Autodesk Inventor part; units mm, degrees
(part 2 of 3)
  line L1096 (95.9721, -65) -> (95.9721, -70)
  line L1097 (107.9721, -65) -> (102.9721, -65)
  line L1098 (100.9721, -70) -> (100.9721, -65)
  line L1099 (102.9721, -65) -> (102.9721, -70)
  line L1100 (107.9721, -70) -> (107.9721, -65)
  line L1101 (102.9721, -70) -> (107.9721, -70)
  line L1102 (114.9721, -65) -> (109.9721, -65)
  line L1103 (109.9721, -65) -> (109.9721, -70)
  line L1104 (109.9721, -70) -> (114.9721, -70)
  line L1105 (114.9721, -70) -> (114.9721, -65)
  line L1106 (116.9721, -65) -> (116.9721, -70)
  line L1107 (128.9721, -65) -> (123.9721, -65)
  line L1108 (128.9721, -70) -> (128.9721, -65)
  line L1109 (123.9721, -70) -> (128.9721, -70)
  line L1110 (121.9721, -65) -> (116.9721, -65)
  line L1111 (121.9721, -70) -> (121.9721, -65)
  line L1112 (116.9721, -70) -> (121.9721, -70)
  line L1113 (123.9721, -65) -> (123.9721, -70)
  line L1114 (142.9721, -65) -> (137.9721, -65)
  line L1115 (137.9721, -70) -> (142.9721, -70)
  line L1116 (142.9721, -70) -> (142.9721, -65)
  line L1117 (137.9721, -65) -> (137.9721, -70)
  line L1118 (135.9721, -65) -> (130.9721, -65)
  line L1119 (135.9721, -70) -> (135.9721, -65)
  line L1120 (130.9721, -65) -> (130.9721, -70)
  line L1121 (130.9721, -70) -> (135.9721, -70)
  line L1122 (156.9721, -14) -> (156.9721, -9)
  line L1123 (156.9721, -9) -> (151.9721, -9)
  line L1124 (151.9721, -14) -> (156.9721, -14)
  line L1125 (151.9721, -9) -> (151.9721, -14)
  line L1126 (156.9721, -16) -> (151.9721, -16)
  line L1127 (151.9721, -21) -> (156.9721, -21)
  line L1128 (156.9721, -21) -> (156.9721, -16)
  line L1129 (151.9721, -16) -> (151.9721, -21)
  line L1130 (151.9721, -23) -> (151.9721, -28)
  line L1131 (156.9721, -23) -> (151.9721, -23)
  line L1132 (151.9721, -28) -> (156.9721, -28)
  line L1133 (156.9721, -28) -> (156.9721, -23)
  line L1134 (151.9721, -30) -> (151.9721, -35)
  line L1135 (156.9721, -30) -> (151.9721, -30)
  line L1136 (151.9721, -35) -> (156.9721, -35)
  line L1137 (156.9721, -35) -> (156.9721, -30)
  line L1138 (151.9721, -37) -> (151.9721, -42)
  line L1139 (156.9721, -37) -> (151.9721, -37)
  line L1140 (151.9721, -42) -> (156.9721, -42)
  line L1141 (156.9721, -42) -> (156.9721, -37)
  line L1142 (151.9721, -44) -> (151.9721, -49)
  line L1143 (156.9721, -44) -> (151.9721, -44)
  line L1144 (151.9721, -49) -> (156.9721, -49)
  line L1145 (156.9721, -49) -> (156.9721, -44)
  line L1146 (151.9721, -51) -> (151.9721, -56)
  line L1147 (156.9721, -51) -> (151.9721, -51)
  line L1148 (151.9721, -56) -> (156.9721, -56)
  line L1149 (156.9721, -56) -> (156.9721, -51)
  line L1150 (163.9721, -14) -> (163.9721, -9)
  line L1151 (163.9721, -9) -> (158.9721, -9)
  line L1152 (158.9721, -9) -> (158.9721, -14)
  line L1153 (158.9721, -14) -> (163.9721, -14)
  line L1154 (163.9721, -16) -> (158.9721, -16)
  line L1155 (158.9721, -21) -> (163.9721, -21)
  line L1156 (163.9721, -21) -> (163.9721, -16)
  line L1157 (158.9721, -16) -> (158.9721, -21)
  line L1158 (163.9721, -23) -> (158.9721, -23)
  line L1159 (158.9721, -23) -> (158.9721, -28)
  line L1160 (158.9721, -28) -> (163.9721, -28)
  line L1161 (163.9721, -28) -> (163.9721, -23)
  line L1162 (163.9721, -30) -> (158.9721, -30)
  line L1163 (158.9721, -30) -> (158.9721, -35)
  line L1164 (158.9721, -35) -> (163.9721, -35)
  line L1165 (163.9721, -35) -> (163.9721, -30)
  line L1166 (158.9721, -44) -> (158.9721, -49)
  line L1167 (163.9721, -49) -> (163.9721, -44)
  line L1168 (163.9721, -44) -> (158.9721, -44)
  line L1169 (158.9721, -42) -> (163.9721, -42)
  line L1170 (163.9721, -42) -> (163.9721, -37)
  line L1171 (163.9721, -37) -> (158.9721, -37)
  line L1172 (158.9721, -37) -> (158.9721, -42)
  line L1173 (158.9721, -49) -> (163.9721, -49)
  line L1174 (172.9721, -9) -> (172.9721, -14)
  line L1175 (172.9721, -14) -> (177.9721, -14)
  line L1176 (177.9721, -14) -> (177.9721, -9)
  line L1177 (177.9721, -9) -> (172.9721, -9)
  line L1178 (109.9721, 65) -> (114.9721, 65)
  line L1179 (116.9721, 65) -> (121.9721, 65)
  line L1180 (114.9721, 70) -> (109.9721, 70)
  line L1181 (114.9721, 65) -> (114.9721, 70)
  line L1182 (116.9721, 70) -> (116.9721, 65)
  line L1183 (121.9721, 70) -> (116.9721, 70)
  line L1184 (121.9721, 65) -> (121.9721, 70)
  line L1185 (109.9721, 70) -> (109.9721, 65)
  line L1186 (107.9721, 65) -> (107.9721, 70)
  line L1187 (102.9721, 65) -> (107.9721, 65)
  line L1188 (107.9721, 70) -> (102.9721, 70)
  line L1189 (102.9721, 70) -> (102.9721, 65)
  line L1190 (88.9721, 65) -> (93.9721, 65)
  line L1191 (95.9721, 70) -> (95.9721, 65)
  line L1192 (100.9721, 70) -> (95.9721, 70)
  line L1193 (93.9721, 65) -> (93.9721, 70)
  line L1194 (93.9721, 70) -> (88.9721, 70)
  line L1195 (100.9721, 65) -> (100.9721, 70)
  line L1196 (95.9721, 65) -> (100.9721, 65)
  line L1197 (88.9721, 70) -> (88.9721, 65)
  line L1198 (86.9721, 65) -> (86.9721, 70)
  line L1199 (81.9721, 65) -> (86.9721, 65)
  line L1200 (81.9721, 70) -> (81.9721, 65)
  line L1201 (86.9721, 70) -> (81.9721, 70)
  line L1202 (67.9721, 65) -> (72.9721, 65)
  line L1203 (67.9721, 70) -> (67.9721, 65)
  line L1204 (72.9721, 70) -> (67.9721, 70)
  line L1205 (74.9721, 65) -> (79.9721, 65)
  line L1206 (72.9721, 65) -> (72.9721, 70)
  line L1207 (74.9721, 70) -> (74.9721, 65)
  line L1208 (79.9721, 65) -> (79.9721, 70)
  line L1209 (79.9721, 70) -> (74.9721, 70)
  line L1210 (123.9721, 65) -> (128.9721, 65)
  line L1211 (128.9721, 70) -> (123.9721, 70)
  line L1212 (123.9721, 70) -> (123.9721, 65)
  line L1213 (128.9721, 65) -> (128.9721, 70)
  line L1214 (130.9721, 65) -> (135.9721, 65)
  line L1215 (130.9721, 70) -> (130.9721, 65)
  line L1216 (135.9721, 65) -> (135.9721, 70)
  line L1217 (137.9721, 70) -> (137.9721, 65)
  line L1218 (135.9721, 70) -> (130.9721, 70)
  line L1219 (137.9721, 65) -> (142.9721, 65)
  line L1220 (142.9721, 70) -> (137.9721, 70)
  line L1221 (142.9721, 65) -> (142.9721, 70)
  line L1222 (53.9721, 70) -> (53.9721, 65)
  line L1223 (58.9721, 70) -> (53.9721, 70)
  line L1224 (53.9721, 65) -> (58.9721, 65)
  line L1225 (58.9721, 65) -> (58.9721, 70)
  line L1226 (60.9721, 70) -> (60.9721, 65)
  line L1227 (65.9721, 70) -> (60.9721, 70)
  line L1228 (60.9721, 65) -> (65.9721, 65)
  line L1229 (65.9721, 65) -> (65.9721, 70)
  line L1230 (39.9721, 70) -> (39.9721, 65)
  line L1231 (44.9721, 70) -> (39.9721, 70)
  line L1232 (44.9721, 65) -> (44.9721, 70)
  line L1233 (46.9721, 70) -> (46.9721, 65)
  line L1234 (46.9721, 65) -> (51.9721, 65)
  line L1235 (51.9721, 65) -> (51.9721, 70)
  line L1236 (51.9721, 70) -> (46.9721, 70)
  line L1237 (39.9721, 65) -> (44.9721, 65)
  line L1238 (102.9721, 77) -> (102.9721, 72)
  line L1239 (100.9721, 72) -> (100.9721, 77)
  line L1240 (95.9721, 72) -> (100.9721, 72)
  line L1241 (100.9721, 77) -> (95.9721, 77)
  line L1242 (93.9721, 77) -> (88.9721, 77)
  line L1243 (93.9721, 72) -> (93.9721, 77)
  line L1244 (95.9721, 77) -> (95.9721, 72)
  line L1245 (88.9721, 72) -> (93.9721, 72)
  line L1246 (88.9721, 77) -> (88.9721, 72)
  line L1247 (81.9721, 72) -> (86.9721, 72)
  line L1248 (86.9721, 72) -> (86.9721, 77)
  line L1249 (86.9721, 77) -> (81.9721, 77)
  line L1250 (72.9721, 72) -> (72.9721, 77)
  line L1251 (74.9721, 77) -> (74.9721, 72)
  line L1252 (79.9721, 77) -> (74.9721, 77)
  line L1253 (79.9721, 72) -> (79.9721, 77)
  line L1254 (81.9721, 77) -> (81.9721, 72)
  line L1255 (74.9721, 72) -> (79.9721, 72)
  line L1256 (67.9721, 77) -> (67.9721, 72)
  line L1257 (72.9721, 77) -> (67.9721, 77)
  line L1258 (67.9721, 72) -> (72.9721, 72)
  line L1259 (65.9721, 72) -> (65.9721, 77)
  line L1260 (60.9721, 72) -> (65.9721, 72)
  line L1261 (60.9721, 77) -> (60.9721, 72)
  line L1262 (65.9721, 77) -> (60.9721, 77)
  line L1263 (58.9721, 77) -> (53.9721, 77)
  line L1264 (58.9721, 72) -> (58.9721, 77)
  line L1265 (53.9721, 72) -> (58.9721, 72)
  line L1266 (53.9721, 77) -> (53.9721, 72)
  line L1267 (123.9721, 72) -> (128.9721, 72)
  line L1268 (128.9721, 77) -> (123.9721, 77)
  line L1269 (123.9721, 77) -> (123.9721, 72)
  line L1270 (116.9721, 72) -> (121.9721, 72)
  line L1271 (121.9721, 72) -> (121.9721, 77)
  line L1272 (121.9721, 77) -> (116.9721, 77)
  line L1273 (116.9721, 77) -> (116.9721, 72)
  line L1274 (114.9721, 72) -> (114.9721, 77)
  line L1275 (109.9721, 72) -> (114.9721, 72)
  line L1276 (114.9721, 77) -> (109.9721, 77)
  line L1277 (102.9721, 72) -> (107.9721, 72)
  line L1278 (109.9721, 77) -> (109.9721, 72)
  line L1279 (107.9721, 72) -> (107.9721, 77)
  line L1280 (107.9721, 77) -> (102.9721, 77)
  line L1281 (128.9721, 72) -> (128.9721, 77)
  line L1282 (109.9721, 79) -> (114.9721, 79)
  line L1283 (114.9721, 79) -> (114.9721, 84)
  line L1284 (114.9721, 84) -> (109.9721, 84)
  line L1285 (102.9721, 79) -> (107.9721, 79)
  line L1286 (107.9721, 79) -> (107.9721, 84)
  line L1287 (102.9721, 84) -> (102.9721, 79)
  line L1288 (107.9721, 84) -> (102.9721, 84)
  line L1289 (109.9721, 84) -> (109.9721, 79)
  line L1290 (88.9721, 79) -> (93.9721, 79)
  line L1291 (93.9721, 84) -> (88.9721, 84)
  line L1292 (95.9721, 79) -> (100.9721, 79)
  line L1293 (93.9721, 79) -> (93.9721, 84)
  line L1294 (95.9721, 84) -> (95.9721, 79)
  line L1295 (100.9721, 84) -> (95.9721, 84)
  line L1296 (100.9721, 79) -> (100.9721, 84)
  line L1297 (81.9721, 79) -> (86.9721, 79)
  line L1298 (88.9721, 84) -> (88.9721, 79)
  line L1299 (86.9721, 79) -> (86.9721, 84)
  line L1300 (86.9721, 84) -> (81.9721, 84)
  line L1301 (81.9721, 84) -> (81.9721, 79)
  line L1302 (67.9721, 84) -> (67.9721, 79)
  line L1303 (72.9721, 84) -> (67.9721, 84)
  line L1304 (67.9721, 79) -> (72.9721, 79)
  line L1305 (74.9721, 79) -> (79.9721, 79)
  line L1306 (72.9721, 79) -> (72.9721, 84)
  line L1307 (79.9721, 84) -> (74.9721, 84)
  line L1308 (79.9721, 79) -> (79.9721, 84)
  line L1309 (74.9721, 84) -> (74.9721, 79)
  line L1310 (170.9721, -14) -> (170.9721, -9)
  line L1311 (170.9721, -21) -> (170.9721, -16)
  line L1312 (165.9721, -14) -> (170.9721, -14)
  line L1313 (165.9721, -9) -> (165.9721, -14)
  line L1314 (170.9721, -16) -> (165.9721, -16)
  line L1315 (170.9721, -9) -> (165.9721, -9)
  line L1316 (165.9721, -16) -> (165.9721, -21)
  line L1317 (165.9721, -23) -> (165.9721, -28)
  line L1318 (170.9721, -28) -> (170.9721, -23)
  line L1319 (170.9721, -23) -> (165.9721, -23)
  line L1320 (165.9721, -21) -> (170.9721, -21)
  line L1321 (165.9721, -30) -> (165.9721, -35)
  line L1322 (165.9721, -28) -> (170.9721, -28)
  line L1323 (170.9721, -30) -> (165.9721, -30)
  line L1324 (165.9721, -35) -> (170.9721, -35)
  line L1325 (170.9721, -35) -> (170.9721, -30)
  line L1326 (121.9721, -72) -> (116.9721, -72)
  line L1327 (116.9721, -77) -> (121.9721, -77)
  line L1328 (121.9721, -77) -> (121.9721, -72)
  line L1329 (123.9721, -72) -> (123.9721, -77)
  line L1330 (128.9721, -72) -> (123.9721, -72)
  line L1331 (128.9721, -77) -> (128.9721, -72)
  line L1332 (123.9721, -77) -> (128.9721, -77)
  line L1333 (114.9721, -72) -> (109.9721, -72)
  line L1334 (109.9721, -77) -> (114.9721, -77)
  line L1335 (114.9721, -77) -> (114.9721, -72)
  line L1336 (116.9721, -72) -> (116.9721, -77)
  line L1337 (100.9721, -77) -> (100.9721, -72)
  line L1338 (107.9721, -72) -> (102.9721, -72)
  line L1339 (102.9721, -72) -> (102.9721, -77)
  line L1340 (102.9721, -77) -> (107.9721, -77)
  line L1341 (107.9721, -77) -> (107.9721, -72)
  line L1342 (109.9721, -72) -> (109.9721, -77)
  line L1343 (95.9721, -77) -> (100.9721, -77)
  line L1344 (95.9721, -72) -> (95.9721, -77)
  line L1345 (100.9721, -72) -> (95.9721, -72)
  line L1346 (114.9721, -84) -> (114.9721, -79)
  line L1347 (114.9721, -79) -> (109.9721, -79)
  line L1348 (109.9721, -84) -> (114.9721, -84)
  line L1349 (107.9721, -79) -> (102.9721, -79)
  line L1350 (109.9721, -79) -> (109.9721, -84)
  line L1351 (107.9721, -84) -> (107.9721, -79)
  line L1352 (102.9721, -84) -> (107.9721, -84)
  line L1353 (102.9721, -79) -> (102.9721, -84)
  line L1354 (100.9721, -84) -> (100.9721, -79)
  line L1355 (100.9721, -79) -> (95.9721, -79)
  line L1356 (95.9721, -84) -> (100.9721, -84)
  line L1357 (95.9721, -79) -> (95.9721, -84)
  dimension "d613" = 2
  dimension "d614" = 5
  dimension "d615" = 5
  dimension "d616" = 82
  dimension "d619" = 7
  dimension "d626" = 7
  dimension "d633" = 7
  dimension "d640" = 7
  dimension "d647" = 7
  dimension "d654" = 7
  dimension "d682" = 9
  dimension "d689" = 7
  dimension "d696" = 7
  dimension "d717" = 7
  dimension "d724" = 7
  dimension "d738" = 7
  dimension "d748" = 7
  dimension "d755" = 7
  dimension "d762" = 7
  dimension "d769" = 7
  dimension "d776" = 7
  dimension "d783" = 7
  constraints: 2712 end point, 14 vertical, 5 horizontal, 2 parallel, 1 perpendicular, 2704 other
  measures "d613" distance between parallel lines of L4 L0
  measures "d614" distance between parallel lines of L2 L0
  measures "d615" distance between parallel lines of L3 L1
  measures "d616" distance between parallel lines of L5 L1
  measures "d619" distance of L0.start L6.start
  measures "d626" distance of L0.start L102.start
  measures "d633" distance of L22.start L110.end
  measures "d640" distance of L400.end L481.end
  measures "d647" distance of L574.start L646.start
  measures "d654" distance of L677.start L724.start
  measures "d682" distance of L62.start L796.start
  measures "d689" distance of L834.end L838.end
  measures "d696" distance of L1081.start L1094.start
  measures "d717" distance of L839.start L1122.end
  measures "d724" distance of L1122.end L1150.end
  measures "d738" distance of L812.end L1174.end
  measures "d748" distance of L739.end L1178.end
  measures "d755" distance of L1187.start L1238.end
  measures "d762" distance of L1274.start L1282.end
  measures "d769" distance of L1150.end L1310.end
  measures "d776" distance of L1110.start L1326.start
  measures "d783" distance of L1333.start L1346.end
extrude "Выдавливание103" cut sketch "Эскиз119" against normal blind 10
sketch "Эскиз120" plane through (-91.9721, 4, 0) normal (0, 1, 0) x (1, 0, 0)
  line L0 (-43.9191, 0) -> (225.9723, 0)
  line L1 (225.9723, 0) -> (225.9723, -109.5505)
  line L2 (225.9723, -109.5505) -> (-43.9191, -109.5505)
  line L3 (-43.9191, -109.5505) -> (-43.9191, 0)
  point P0 (91.9721, 0)
  constraints: 8 end point, 2 parallel, 1 horizontal, 1 perpendicular
extrude "Выдавливание104" cut sketch "Эскиз120" against normal through all
mirror "Зеркальное отражение8" about plane through (-46.203, 1.9857, 0) normal (0, 0, 1)
sketch "Эскиз121" plane through (0, 0, 0) normal (0, -1, 0) x (1, 0, 0)
  line L0 (-10, -10) -> (10, -10)
  line L1 (10, -10) -> (10, 10)
  line L2 (10, 10) -> (-10, 10)
  line L3 (-10, 10) -> (-10, -10)
  line L4 (-10, -10) -> (10, 10) construction
  line L5 (10, -10) -> (-10, 10) construction
  point P0 (0, 0)
  dimension "d790" = 20
  dimension "d791" = 20
  constraints: 12 end point, 2 collinear, 2 midpoint, 1 perpendicular, 1 vertical
  measures "d790" distance of L2.end L1.end
  measures "d791" distance of L1.end L0.end
extrude "Выдавливание105" add sketch "Эскиз121" against normal up to surface (4 mm away)
extrude "Выдавливание106" add sketch "Эскиз121" along normal blind 5
sketch "Эскиз122" plane through (0, -5, 0) normal (0, -1, 0) x (1, 0, 0)
  line L0 (-7.5, -7.5) -> (7.5, -7.5)
  line L1 (7.5, -7.5) -> (7.5, 7.5)
  line L2 (7.5, 7.5) -> (-7.5, 7.5)
  line L3 (-7.5, 7.5) -> (-7.5, -7.5)
  line L4 (-7.5, -7.5) -> (7.5, 7.5) construction
  line L5 (7.5, -7.5) -> (-7.5, 7.5) construction
  point P0 (0, 0)
  dimension "d796" = 15
  dimension "d797" = 15
  dimension "d12" = 100
  dimension "d14" = 17
  dimension "d26" = 5
  constraints: 12 end point, 2 midpoint, 2 parallel, 1 horizontal, 1 perpendicular
  measures "d796" distance of L2.end L1.end
  measures "d797" distance of L1.end L0.end
extrude "Выдавливание107" cut sketch "Эскиз122" against normal blind 3
sketch "Эскиз6" plane through (0, -35, -85) normal (0, -1, 0) x (1, 0, 0)
  arc A0 (29.3991, 164.4544) -> (0, 170) centre (-5, 62.7941) ccw projected
  line L0 (0, 170) -> (0, 0) projected
  arc A1 (0, 0) -> (29.3991, 5.5456) centre (-5, 107.2059) ccw projected
  arc A2 (29.3991, 5.5456) -> (100, 85) centre (-5, 107.2059) ccw projected
  arc A3 (100, 85) -> (29.3991, 164.4544) centre (-5, 62.7941) ccw projected
  point P0 (0, 85)
  dimension "d121" = 143.8029
  constraints: 4 end point, 2 point on circle, 1 centre point, 1 coincident, 1 horizontal, 1 vertical
  measures "d121" radius of A0
sketch "Эскиз26" plane through (0, -165, -85) normal (0, -1, 0) x (1, 0, 0)
  arc A0 (97.9549, 85) -> (2, 167.8837) centre (-5, 62.7941) ccw projected
  line L0 (97.9395, 85) -> (97.9395, 85) construction
  line L1 (32, 161.4035) -> (32, 85)
  line L2 (2, 85) -> (100, 85) construction
  line L3 (2, 0.112) -> (2, 167.8837) construction
  line L4 (34, 160.6298) -> (34, 85)
  line L5 (32, 85) -> (34, 85)
  point P0 (0, 85)
  point P1 (2, 22)
  dimension "d144" = 30
  dimension "d145" = 2
  constraints: 6 end point, 2 point on circle, 2 point on line, 1 horizontal, 1 perpendicular, 1 vertical
  measures "d144" distance between parallel lines of L1 L3
  measures "d145" distance between parallel lines of L4 L1
sketch "Эскиз28" plane through (34, -165, 75.6298) normal (1, 0, 0) x (0, 0, -1)
  circle A0 centre (68.6298, 7) radius 5 projected
  line L0 (75.6298, 0) -> (75.6298, 230.325) projected
  line L1 (75.6298, 0) -> (-0.7738, 0) projected
  line L2 (75.6298, 14) -> (61.6298, 14) construction
  line L3 (61.6298, 14) -> (61.6298, 0) construction
  line L4 (160.5178, 0) -> (-7.2539, 0) projected
  line L5 (72.6298, 17) -> (65.6298, 17)
  line L6 (65.6298, 17) -> (65.6298, 27)
  line L7 (65.6298, 27) -> (72.6298, 27)
  line L8 (72.6298, 27) -> (72.6298, 17)
  point P0 (75.6298, 165)
  point P1 (138.6298, 0)
  dimension "d156" = 14
  dimension "d157" = 14
  dimension "d158" = 7
  dimension "d159" = 10
  dimension "d160" = 3
  dimension "d161" = 3
  constraints: 12 end point, 2 horizontal, 2 parallel, 2 perpendicular, 2 point on line
  measures "d156" distance of L0.start L2.start
  measures "d157" distance of L2.start L2.end
  measures "d158" distance of L6.end L7.end
  measures "d159" distance of L5.end L6.end
  measures "d160" distance between parallel lines of L2 L5
  measures "d161" distance between parallel lines of L0 L8
sketch "Эскиз29" plane through (34, -165, 75.6298) normal (1, 0, 0) x (0, 0, -1)
  circle A0 centre (68.6298, 7) radius 5 projected
  line L0 (75.6298, 0) -> (-0.7738, 0) projected
  line L1 (75.6298, 0) -> (75.6298, 230.325) projected
  line L2 (75.6298, 14) -> (61.6298, 14)
  line L3 (61.6298, 14) -> (61.6298, 0)
  line L4 (-9.3702, 0) -> (160.6298, 0) projected
  line L5 (58.6298, 2) -> (51.6298, 2)
  line L6 (51.6298, 2) -> (51.6298, 12)
  line L7 (51.6298, 12) -> (58.6298, 12)
  line L8 (58.6298, 12) -> (58.6298, 2)
  line L9 (65.6298, 17) -> (72.6298, 17) projected
  point P0 (75.6298, 165)
  dimension "d164" = 14
  dimension "d165" = 14
  dimension "d166" = 3
  dimension "d167" = 2
  dimension "d168" = 7
  dimension "d169" = 10
  constraints: 12 end point, 2 horizontal, 2 parallel, 2 perpendicular, 2 point on line
  measures "d164" distance of L2.end L3.end
  measures "d165" distance of L2.start L2.end
  measures "d166" distance between parallel lines of L3 L8
  measures "d167" distance between parallel lines of L0 L5
  measures "d168" distance of L6.end L7.end
  measures "d169" distance of L6.end L5.end
sketch "Эскиз30" plane through (34, -165, 75.6298) normal (1, 0, 0) x (0, 0, -1)
  line L0 (51.6298, 12) -> (51.6298, 2) projected
  line L1 (58.6298, 12) -> (51.6298, 12) projected
  line L2 (58.6298, 2) -> (58.6298, 12) projected
  line L3 (51.6298, 2) -> (58.6298, 2) projected
  line L4 (39.6298, 12) -> (39.6298, 2)
  line L5 (46.6298, 12) -> (39.6298, 12)
  line L6 (46.6298, 2) -> (46.6298, 12)
  line L7 (39.6298, 2) -> (46.6298, 2)
  point P0 (75.6298, 165)
  point P1 (43.1298, 2)
  dimension "d178" = 7
  dimension "d179" = 10
  dimension "d180" = 5
  constraints: 8 end point, 1 horizontal, 1 horizontal alignment, 1 midpoint, 1 vertical
  measures "d178" distance between parallel lines of L4 L6
  measures "d179" distance between parallel lines of L7 L5
  measures "d180" distance between parallel lines of L6 L0
sketch "Эскиз31" plane through (34, -165, 75.6298) normal (1, 0, 0) x (0, 0, -1)
  line L0 (46.6298, 12) -> (39.6298, 12) projected
  line L1 (39.6298, 12) -> (39.6298, 2) projected
  line L2 (46.6298, 2) -> (46.6298, 12) projected
  line L3 (39.6298, 2) -> (46.6298, 2) projected
  line L4 (34.6298, 12) -> (27.6298, 12)
  line L5 (27.6298, 12) -> (27.6298, 2)
  line L6 (34.6298, 2) -> (34.6298, 12)
  line L7 (27.6298, 2) -> (34.6298, 2)
  point P0 (75.6298, 165)
  dimension "d186" = 10
  dimension "d187" = 7
  dimension "d188" = 5
  constraints: 8 end point, 2 horizontal, 2 vertical, 1 horizontal alignment
  measures "d186" distance of L6.start L4.start
  measures "d187" distance of L4.start L4.end
  measures "d188" distance between parallel lines of L1 L6
sketch "Эскиз32" plane through (34, -165, 75.6298) normal (1, 0, 0) x (0, 0, -1)
  line L0 (34.6298, 12) -> (27.6298, 12) projected
  line L1 (27.6298, 12) -> (27.6298, 2) projected
  line L2 (34.6298, 2) -> (34.6298, 12) projected
  line L3 (27.6298, 2) -> (34.6298, 2) projected
  line L4 (22.6298, 12) -> (15.6298, 12)
  line L5 (15.6298, 12) -> (15.6298, 2)
  line L6 (22.6298, 2) -> (22.6298, 12)
  line L7 (15.6298, 2) -> (22.6298, 2)
  point P0 (75.6298, 165)
  dimension "d194" = 10
  dimension "d195" = 7
  dimension "d196" = 5
  constraints: 8 end point, 2 horizontal, 2 vertical, 1 horizontal alignment
  measures "d194" distance of L6.start L4.start
  measures "d195" distance of L4.start L4.end
  measures "d196" distance between parallel lines of L6 L1
sketch "Эскиз33" plane through (34, -165, 75.6298) normal (1, 0, 0) x (0, 0, -1)
  line L0 (22.6298, 12) -> (15.6298, 12) projected
  line L1 (15.6298, 12) -> (15.6298, 2) projected
  line L2 (22.6298, 2) -> (22.6298, 12) projected
  line L3 (15.6298, 2) -> (22.6298, 2) projected
  line L4 (10.6298, 12) -> (3.6298, 12)
  line L5 (3.6298, 12) -> (3.6298, 2)
  line L6 (10.6298, 2) -> (10.6298, 12)
  line L7 (3.6298, 2) -> (10.6298, 2)
  point P0 (75.6298, 165)
  dimension "d202" = 10
  dimension "d203" = 7
  dimension "d204" = 5
  constraints: 8 end point, 2 horizontal, 2 vertical, 1 horizontal alignment
  measures "d202" distance of L6.start L4.start
  measures "d203" distance of L4.start L4.end
  measures "d204" distance between parallel lines of L1 L6
sketch "Эскиз109" plane through (34, -165, 75.6298) normal (1, 0, 0) x (0, 0, -1)
  line L0 (75.6298, 130) -> (75.6298, 245.5199) projected
  line L1 (138.6298, 0) -> (138.6298, 129) projected
  line L2 (138.6298, 129) -> (140.6298, 129) projected
  line L3 (140.6298, 129) -> (150.1813, 129) projected
  line L4 (145.6298, 129) -> (151.2595, 129) projected
  line L5 (152.0333, 129) -> (158.5134, 129) projected
  line L6 (158.5134, 129) -> (75.6298, 129)
  line L7 (75.6298, 129) -> (75.6298, 245.5199)
  line L8 (75.6298, 245.5199) -> (158.5134, 245.5199)
  line L9 (158.5134, 245.5199) -> (158.5134, 129)
  line L10 (138.6298, 129) -> (158.5134, 129)
  line L11 (158.5134, 129) -> (158.5134, 0)
  line L12 (158.5134, 0) -> (138.6298, 0)
  line L13 (138.6298, 0) -> (138.6298, 129)
  point P0 (75.6298, 165)
  constraints: 16 end point, 4 parallel, 2 horizontal, 2 perpendicular
sketch "Эскиз110" plane through (34, -165, 75.6298) normal (1, 0, 0) x (0, 0, -1)
  line L0 (85.6298, 122) -> (78.6298, 122) projected
  line L1 (135.6298, 122) -> (128.6298, 122) projected
  line L2 (75.6298, 129) -> (138.6298, 129)
  line L3 (138.6298, 129) -> (138.6298, 122)
  line L4 (138.6298, 122) -> (75.6298, 122)
  line L5 (75.6298, 122) -> (75.6298, 129)
  point P0 (75.6298, 165)
  point P1 (78.6298, 129)
  constraints: 8 end point, 2 parallel, 1 coincident, 1 horizontal, 1 perpendicular, 1 point on line
sketch "Эскиз111" plane through (34, -165, 75.6298) normal (1, 0, 0) x (0, 0, -1)
  line L0 (128.6298, 117) -> (128.6298, 107) construction
  line L1 (128.6298, 107) -> (135.6298, 107) construction
  line L2 (135.6298, 107) -> (135.6298, 117) construction
  line L3 (135.6298, 117) -> (128.6298, 117) construction
  line L4 (128.6298, 102) -> (128.6298, 92) construction
  line L5 (128.6298, 92) -> (135.6298, 92) construction
  line L6 (135.6298, 92) -> (135.6298, 102) construction
  line L7 (135.6298, 102) -> (128.6298, 102) construction
  line L8 (128.6298, 87) -> (128.6298, 77) construction
  line L9 (128.6298, 77) -> (135.6298, 77) construction
  line L10 (135.6298, 77) -> (135.6298, 87) construction
  line L11 (135.6298, 87) -> (128.6298, 87) construction
  line L12 (128.6298, 72) -> (128.6298, 62) construction
  line L13 (128.6298, 62) -> (135.6298, 62) construction
  line L14 (135.6298, 62) -> (135.6298, 72) construction
  line L15 (135.6298, 72) -> (128.6298, 72) construction
  line L16 (128.6298, 57) -> (128.6298, 47) construction
  line L17 (128.6298, 47) -> (135.6298, 47) construction
  line L18 (135.6298, 47) -> (135.6298, 57) construction
  line L19 (135.6298, 57) -> (128.6298, 57) construction
  line L20 (128.6298, 42) -> (128.6298, 32) construction
  line L21 (128.6298, 32) -> (135.6298, 32) construction
  line L22 (135.6298, 32) -> (135.6298, 42) construction
  line L23 (135.6298, 42) -> (128.6298, 42) construction
  line L24 (128.6298, 27) -> (128.6298, 17) construction
  line L25 (128.6298, 17) -> (135.6298, 17) construction
  line L26 (135.6298, 17) -> (135.6298, 27) construction
  line L27 (135.6298, 27) -> (128.6298, 27) construction
  line L28 (128.6298, 12) -> (128.6298, 2) construction
  line L29 (128.6298, 2) -> (135.6298, 2) construction
  line L30 (135.6298, 2) -> (135.6298, 12) construction
  line L31 (135.6298, 12) -> (128.6298, 12) construction
  line L32 (116.6298, 117) -> (116.6298, 107) construction
  line L33 (116.6298, 107) -> (123.6298, 107) construction
  line L34 (123.6298, 107) -> (123.6298, 117) construction
  line L35 (123.6298, 117) -> (116.6298, 117) construction
  line L36 (116.6298, 102) -> (116.6298, 92) construction
  line L37 (116.6298, 92) -> (123.6298, 92) construction
  line L38 (123.6298, 92) -> (123.6298, 102) construction
  line L39 (123.6298, 102) -> (116.6298, 102) construction
  line L40 (116.6298, 87) -> (116.6298, 77) construction
  line L41 (116.6298, 77) -> (123.6298, 77) construction
  line L42 (123.6298, 77) -> (123.6298, 87) construction
  line L43 (123.6298, 87) -> (116.6298, 87) construction
  line L44 (116.6298, 72) -> (116.6298, 62) construction
  line L45 (116.6298, 62) -> (123.6298, 62) construction
  line L46 (123.6298, 62) -> (123.6298, 72) construction
  line L47 (123.6298, 72) -> (116.6298, 72) construction
  line L48 (116.6298, 57) -> (116.6298, 47) construction
  line L49 (116.6298, 47) -> (123.6298, 47) construction
  line L50 (123.6298, 47) -> (123.6298, 57) construction
  line L51 (123.6298, 57) -> (116.6298, 57) construction
  line L52 (116.6298, 42) -> (116.6298, 32) construction
  line L53 (116.6298, 32) -> (123.6298, 32) construction
  line L54 (123.6298, 32) -> (123.6298, 42) construction
  line L55 (123.6298, 42) -> (116.6298, 42) construction
  line L56 (116.6298, 27) -> (116.6298, 17) construction
  line L57 (116.6298, 17) -> (123.6298, 17) construction
  line L58 (123.6298, 17) -> (123.6298, 27) construction
  line L59 (123.6298, 27) -> (116.6298, 27) construction
  line L60 (116.6298, 12) -> (116.6298, 2) construction
  line L61 (116.6298, 2) -> (123.6298, 2) construction
  line L62 (123.6298, 2) -> (123.6298, 12) construction
  line L63 (123.6298, 12) -> (116.6298, 12) construction
  line L64 (111.6298, 117) -> (104.6298, 117) construction
  line L65 (104.6298, 117) -> (104.6298, 107) construction
  line L66 (104.6298, 107) -> (111.6298, 107) construction
  line L67 (111.6298, 107) -> (111.6298, 117) construction
  line L68 (111.6298, 102) -> (104.6298, 102) construction
  line L69 (104.6298, 102) -> (104.6298, 92) construction
  line L70 (104.6298, 92) -> (111.6298, 92) construction
  line L71 (111.6298, 92) -> (111.6298, 102) construction
  line L72 (111.6298, 87) -> (104.6298, 87) construction
  line L73 (104.6298, 87) -> (104.6298, 77) construction
  line L74 (104.6298, 77) -> (111.6298, 77) construction
  line L75 (111.6298, 77) -> (111.6298, 87) construction
  line L76 (111.6298, 72) -> (104.6298, 72) construction
  line L77 (104.6298, 72) -> (104.6298, 62) construction
  line L78 (104.6298, 62) -> (111.6298, 62) construction
  line L79 (111.6298, 62) -> (111.6298, 72) construction
  line L80 (111.6298, 57) -> (104.6298, 57) construction
  line L81 (104.6298, 57) -> (104.6298, 47) construction
  line L82 (104.6298, 47) -> (111.6298, 47) construction
  line L83 (111.6298, 47) -> (111.6298, 57) construction
  line L84 (111.6298, 42) -> (104.6298, 42) construction
  line L85 (104.6298, 42) -> (104.6298, 32) construction
  line L86 (104.6298, 32) -> (111.6298, 32) construction
  line L87 (111.6298, 32) -> (111.6298, 42) construction
  line L88 (111.6298, 27) -> (104.6298, 27) construction
  line L89 (104.6298, 27) -> (104.6298, 17) construction
  line L90 (104.6298, 17) -> (111.6298, 17) construction
  line L91 (111.6298, 17) -> (111.6298, 27) construction
  line L92 (65.6298, 27) -> (65.6298, 17) construction
  line L93 (65.6298, 17) -> (72.6298, 17) construction
  line L94 (72.6298, 17) -> (72.6298, 27) construction
  line L95 (72.6298, 27) -> (65.6298, 27) construction
  line L96 (51.6298, 12) -> (51.6298, 2) construction
  line L97 (51.6298, 2) -> (58.6298, 2) construction
  line L98 (58.6298, 2) -> (58.6298, 12) construction
  line L99 (58.6298, 12) -> (51.6298, 12) construction
  line L100 (51.6298, 27) -> (51.6298, 17) construction
  line L101 (51.6298, 17) -> (58.6298, 17) construction
  line L102 (58.6298, 17) -> (58.6298, 27) construction
  line L103 (58.6298, 27) -> (51.6298, 27) construction
  line L104 (51.6298, 42) -> (51.6298, 32) construction
  line L105 (51.6298, 32) -> (58.6298, 32) construction
  line L106 (58.6298, 32) -> (58.6298, 42) construction
  line L107 (58.6298, 42) -> (51.6298, 42) construction
  line L108 (51.6298, 57) -> (51.6298, 47) construction
  line L109 (51.6298, 47) -> (58.6298, 47) construction
  line L110 (58.6298, 47) -> (58.6298, 57) construction
  line L111 (58.6298, 57) -> (51.6298, 57) construction
  line L112 (51.6298, 72) -> (51.6298, 62) construction
  line L113 (51.6298, 62) -> (58.6298, 62) construction
  line L114 (58.6298, 62) -> (58.6298, 72) construction
  line L115 (58.6298, 72) -> (51.6298, 72) construction
  line L116 (51.6298, 87) -> (51.6298, 77) construction
  line L117 (51.6298, 77) -> (58.6298, 77) construction
  line L118 (58.6298, 77) -> (58.6298, 87) construction
  line L119 (58.6298, 87) -> (51.6298, 87) construction
  line L120 (51.6298, 102) -> (51.6298, 92) construction
  line L121 (51.6298, 92) -> (58.6298, 92) construction
  line L122 (58.6298, 92) -> (58.6298, 102) construction
  line L123 (58.6298, 102) -> (51.6298, 102) construction
  line L124 (51.6298, 117) -> (51.6298, 107) construction
  line L125 (51.6298, 107) -> (58.6298, 107) construction
  line L126 (58.6298, 107) -> (58.6298, 117) construction
  line L127 (58.6298, 117) -> (51.6298, 117) construction
  line L128 (51.6298, 132) -> (51.6298, 122) construction
  line L129 (51.6298, 122) -> (58.6298, 122) construction
  line L130 (58.6298, 122) -> (58.6298, 132) construction
  line L131 (58.6298, 132) -> (51.6298, 132) construction
  line L132 (51.6298, 147) -> (51.6298, 137) construction
  line L133 (51.6298, 137) -> (58.6298, 137) construction
  line L134 (58.6298, 137) -> (58.6298, 147) construction
  line L135 (58.6298, 147) -> (51.6298, 147) construction
  line L136 (51.6298, 162) -> (51.6298, 152) construction
  line L137 (51.6298, 152) -> (58.6298, 152) construction
  line L138 (58.6298, 152) -> (58.6298, 162) construction
  line L139 (58.6298, 162) -> (51.6298, 162) construction
  line L140 (51.6298, 177) -> (51.6298, 167) construction
  line L141 (51.6298, 167) -> (58.6298, 167) construction
  line L142 (58.6298, 167) -> (58.6298, 177) construction
  line L143 (58.6298, 177) -> (51.6298, 177) construction
  line L144 (51.6298, 192) -> (51.6298, 182) construction
  line L145 (51.6298, 182) -> (58.6298, 182) construction
  line L146 (58.6298, 182) -> (58.6298, 192) construction
  line L147 (58.6298, 192) -> (51.6298, 192) construction
  line L148 (51.6298, 207) -> (51.6298, 197) construction
  line L149 (51.6298, 197) -> (58.6298, 197) construction
  line L150 (58.6298, 197) -> (58.6298, 207) construction
  line L151 (58.6298, 207) -> (51.6298, 207) construction
  line L152 (51.6298, 222) -> (51.6298, 212) construction
  line L153 (51.6298, 212) -> (58.6298, 212) construction
  line L154 (58.6298, 212) -> (58.6298, 222) construction
  line L155 (58.6298, 222) -> (51.6298, 222) construction
  line L156 (65.6298, 42) -> (65.6298, 32) construction
  line L157 (65.6298, 32) -> (72.6298, 32) construction
  line L158 (72.6298, 32) -> (72.6298, 42) construction
  line L159 (72.6298, 42) -> (65.6298, 42) construction
  line L160 (65.6298, 57) -> (65.6298, 47) construction
  line L161 (65.6298, 47) -> (72.6298, 47) construction
  line L162 (72.6298, 47) -> (72.6298, 57) construction
  line L163 (72.6298, 57) -> (65.6298, 57) construction
  line L164 (65.6298, 72) -> (65.6298, 62) construction
  line L165 (65.6298, 62) -> (72.6298, 62) construction
  line L166 (72.6298, 62) -> (72.6298, 72) construction
  line L167 (72.6298, 72) -> (65.6298, 72) construction
  line L168 (65.6298, 87) -> (65.6298, 77) construction
  line L169 (65.6298, 77) -> (72.6298, 77) construction
  line L170 (72.6298, 77) -> (72.6298, 87) construction
  line L171 (72.6298, 87) -> (65.6298, 87) construction
  line L172 (65.6298, 102) -> (65.6298, 92) construction
  line L173 (65.6298, 92) -> (72.6298, 92) construction
  line L174 (72.6298, 92) -> (72.6298, 102) construction
  line L175 (72.6298, 102) -> (65.6298, 102) construction
  line L176 (65.6298, 117) -> (65.6298, 107) construction
  line L177 (65.6298, 107) -> (72.6298, 107) construction
  line L178 (72.6298, 107) -> (72.6298, 117) construction
  line L179 (72.6298, 117) -> (65.6298, 117) construction
  line L180 (65.6298, 132) -> (65.6298, 122) construction
  line L181 (65.6298, 122) -> (72.6298, 122) construction
  line L182 (72.6298, 122) -> (72.6298, 132) construction
  line L183 (72.6298, 132) -> (65.6298, 132) construction
  line L184 (65.6298, 147) -> (65.6298, 137) construction
  line L185 (65.6298, 137) -> (72.6298, 137) construction
  line L186 (72.6298, 137) -> (72.6298, 147) construction
  line L187 (72.6298, 147) -> (65.6298, 147) construction
  line L188 (65.6298, 162) -> (65.6298, 152) construction
  line L189 (65.6298, 152) -> (72.6298, 152) construction
  line L190 (72.6298, 152) -> (72.6298, 162) construction
  line L191 (72.6298, 162) -> (65.6298, 162) construction
  line L192 (65.6298, 177) -> (65.6298, 167) construction
  line L193 (65.6298, 167) -> (72.6298, 167) construction
  line L194 (72.6298, 167) -> (72.6298, 177) construction
  line L195 (72.6298, 177) -> (65.6298, 177) construction
  line L196 (65.6298, 192) -> (65.6298, 182) construction
  line L197 (65.6298, 182) -> (72.6298, 182) construction
  line L198 (72.6298, 182) -> (72.6298, 192) construction
  line L199 (72.6298, 192) -> (65.6298, 192) construction
  line L200 (65.6298, 207) -> (65.6298, 197) construction
  line L201 (65.6298, 197) -> (72.6298, 197) construction
  line L202 (72.6298, 197) -> (72.6298, 207) construction
  line L203 (72.6298, 207) -> (65.6298, 207) construction
  line L204 (65.6298, 222) -> (65.6298, 212) construction
  line L205 (65.6298, 212) -> (72.6298, 212) construction
  line L206 (72.6298, 212) -> (72.6298, 222) construction
  line L207 (72.6298, 222) -> (65.6298, 222) construction
  line L208 (46.6298, 27) -> (39.6298, 27) construction
  line L209 (39.6298, 27) -> (39.6298, 17) construction
  line L210 (39.6298, 17) -> (46.6298, 17) construction
  line L211 (46.6298, 17) -> (46.6298, 27) construction
  line L212 (46.6298, 42) -> (39.6298, 42) construction
  line L213 (39.6298, 42) -> (39.6298, 32) construction
  line L214 (39.6298, 32) -> (46.6298, 32) construction
  line L215 (46.6298, 32) -> (46.6298, 42) construction
  line L216 (46.6298, 57) -> (39.6298, 57) construction
  line L217 (39.6298, 57) -> (39.6298, 47) construction
  line L218 (39.6298, 47) -> (46.6298, 47) construction
  line L219 (46.6298, 47) -> (46.6298, 57) construction
  line L220 (46.6298, 72) -> (39.6298, 72) construction
  line L221 (39.6298, 72) -> (39.6298, 62) construction
  line L222 (39.6298, 62) -> (46.6298, 62) construction
  line L223 (46.6298, 62) -> (46.6298, 72) construction
  line L224 (46.6298, 87) -> (39.6298, 87) construction
  line L225 (39.6298, 87) -> (39.6298, 77) construction
  line L226 (39.6298, 77) -> (46.6298, 77) construction
  line L227 (46.6298, 77) -> (46.6298, 87) construction
  line L228 (46.6298, 102) -> (39.6298, 102) construction
  line L229 (39.6298, 102) -> (39.6298, 92) construction
  line L230 (39.6298, 92) -> (46.6298, 92) construction
  line L231 (46.6298, 92) -> (46.6298, 102) construction
  line L232 (46.6298, 117) -> (39.6298, 117) construction
  line L233 (39.6298, 117) -> (39.6298, 107) construction
  line L234 (39.6298, 107) -> (46.6298, 107) construction
  line L235 (46.6298, 107) -> (46.6298, 117) construction
  line L236 (46.6298, 132) -> (39.6298, 132) construction
  line L237 (39.6298, 132) -> (39.6298, 122) construction
  line L238 (39.6298, 122) -> (46.6298, 122) construction
  line L239 (46.6298, 122) -> (46.6298, 132) construction
  line L240 (46.6298, 147) -> (39.6298, 147) construction
  line L241 (39.6298, 147) -> (39.6298, 137) construction
  line L242 (39.6298, 137) -> (46.6298, 137) construction
  line L243 (46.6298, 137) -> (46.6298, 147) construction
  line L244 (46.6298, 162) -> (39.6298, 162) construction
  line L245 (39.6298, 162) -> (39.6298, 152) construction
  line L246 (39.6298, 152) -> (46.6298, 152) construction
  line L247 (46.6298, 152) -> (46.6298, 162) construction
  line L248 (46.6298, 177) -> (39.6298, 177) construction
  line L249 (39.6298, 177) -> (39.6298, 167) construction
  line L250 (39.6298, 167) -> (46.6298, 167) construction
  line L251 (46.6298, 167) -> (46.6298, 177) construction
  line L252 (46.6298, 192) -> (39.6298, 192) construction
  line L253 (39.6298, 192) -> (39.6298, 182) construction
  line L254 (39.6298, 182) -> (46.6298, 182) construction
  line L255 (46.6298, 182) -> (46.6298, 192) construction
  line L256 (46.6298, 207) -> (39.6298, 207) construction
  line L257 (39.6298, 207) -> (39.6298, 197) construction
  line L258 (39.6298, 197) -> (46.6298, 197) construction
  line L259 (46.6298, 197) -> (46.6298, 207) construction
  line L260 (34.6298, 2) -> (34.6298, 12) construction
  line L261 (34.6298, 12) -> (27.6298, 12) construction
  line L262 (27.6298, 12) -> (27.6298, 2) construction
  line L263 (27.6298, 2) -> (34.6298, 2) construction
  line L264 (34.6298, 17) -> (34.6298, 27) construction
  line L265 (34.6298, 27) -> (27.6298, 27) construction
  line L266 (27.6298, 27) -> (27.6298, 17) construction
  line L267 (27.6298, 17) -> (34.6298, 17) construction
  line L268 (34.6298, 32) -> (34.6298, 42) construction
  line L269 (34.6298, 42) -> (27.6298, 42) construction
  line L270 (27.6298, 42) -> (27.6298, 32) construction
  line L271 (27.6298, 32) -> (34.6298, 32) construction
  line L272 (34.6298, 47) -> (34.6298, 57) construction
  line L273 (34.6298, 57) -> (27.6298, 57) construction
  line L274 (27.6298, 57) -> (27.6298, 47) construction
  line L275 (27.6298, 47) -> (34.6298, 47) construction
  line L276 (34.6298, 62) -> (34.6298, 72) construction
  line L277 (34.6298, 72) -> (27.6298, 72) construction
  line L278 (27.6298, 72) -> (27.6298, 62) construction
  line L279 (27.6298, 62) -> (34.6298, 62) construction
  line L280 (34.6298, 77) -> (34.6298, 87) construction
  line L281 (34.6298, 87) -> (27.6298, 87) construction
  line L282 (27.6298, 87) -> (27.6298, 77) construction
  line L283 (27.6298, 77) -> (34.6298, 77) construction
  line L284 (34.6298, 92) -> (34.6298, 102) construction
  line L285 (34.6298, 102) -> (27.6298, 102) construction
  line L286 (27.6298, 102) -> (27.6298, 92) construction
  line L287 (27.6298, 92) -> (34.6298, 92) construction
  line L288 (34.6298, 107) -> (34.6298, 117) construction
  line L289 (34.6298, 117) -> (27.6298, 117) construction
  line L290 (27.6298, 117) -> (27.6298, 107) construction
  line L291 (27.6298, 107) -> (34.6298, 107) construction
  line L292 (34.6298, 122) -> (34.6298, 132) construction
  line L293 (34.6298, 132) -> (27.6298, 132) construction
  line L294 (27.6298, 132) -> (27.6298, 122) construction
  line L295 (27.6298, 122) -> (34.6298, 122) construction
  line L296 (34.6298, 137) -> (34.6298, 147) construction
  line L297 (34.6298, 147) -> (27.6298, 147) construction
  line L298 (27.6298, 147) -> (27.6298, 137) construction
  line L299 (27.6298, 137) -> (34.6298, 137) construction
  line L300 (34.6298, 152) -> (34.6298, 162) construction
  line L301 (34.6298, 162) -> (27.6298, 162) construction
  line L302 (27.6298, 162) -> (27.6298, 152) construction
  line L303 (27.6298, 152) -> (34.6298, 152) construction
  line L304 (34.6298, 167) -> (34.6298, 177) construction
  line L305 (34.6298, 177) -> (27.6298, 177) construction
  line L306 (27.6298, 177) -> (27.6298, 167) construction
  line L307 (27.6298, 167) -> (34.6298, 167) construction
  line L308 (34.6298, 182) -> (34.6298, 192) construction
  line L309 (34.6298, 192) -> (27.6298, 192) construction
  line L310 (27.6298, 192) -> (27.6298, 182) construction
  line L311 (27.6298, 182) -> (34.6298, 182) construction
  line L312 (34.6298, 197) -> (34.6298, 207) construction
  line L313 (34.6298, 207) -> (27.6298, 207) construction
  line L314 (27.6298, 207) -> (27.6298, 197) construction
  line L315 (27.6298, 197) -> (34.6298, 197) construction
  line L316 (22.6298, 2) -> (22.6298, 12) construction
  line L317 (22.6298, 12) -> (15.6298, 12) construction
  line L318 (15.6298, 12) -> (15.6298, 2) construction
  line L319 (15.6298, 2) -> (22.6298, 2) construction
  line L320 (22.6298, 17) -> (22.6298, 27) construction
  line L321 (22.6298, 27) -> (15.6298, 27) construction
  line L322 (15.6298, 27) -> (15.6298, 17) construction
  line L323 (15.6298, 17) -> (22.6298, 17) construction
  line L324 (22.6298, 32) -> (22.6298, 42) construction
  line L325 (22.6298, 42) -> (15.6298, 42) construction
  line L326 (15.6298, 42) -> (15.6298, 32) construction
  line L327 (15.6298, 32) -> (22.6298, 32) construction
  line L328 (22.6298, 47) -> (22.6298, 57) construction
  line L329 (22.6298, 57) -> (15.6298, 57) construction
  line L330 (15.6298, 57) -> (15.6298, 47) construction
  line L331 (15.6298, 47) -> (22.6298, 47) construction
  line L332 (22.6298, 62) -> (22.6298, 72) construction
  line L333 (22.6298, 72) -> (15.6298, 72) construction
  line L334 (15.6298, 72) -> (15.6298, 62) construction
  line L335 (15.6298, 62) -> (22.6298, 62) construction
  line L336 (22.6298, 77) -> (22.6298, 87) construction
  line L337 (22.6298, 87) -> (15.6298, 87) construction
  line L338 (15.6298, 87) -> (15.6298, 77) construction
  line L339 (15.6298, 77) -> (22.6298, 77) construction
  line L340 (22.6298, 92) -> (22.6298, 102) construction
  line L341 (22.6298, 102) -> (15.6298, 102) construction
  line L342 (15.6298, 102) -> (15.6298, 92) construction
  line L343 (15.6298, 92) -> (22.6298, 92) construction
  line L344 (22.6298, 107) -> (22.6298, 117) construction
  line L345 (22.6298, 117) -> (15.6298, 117) construction
  line L346 (15.6298, 117) -> (15.6298, 107) construction
  line L347 (15.6298, 107) -> (22.6298, 107) construction
  line L348 (22.6298, 122) -> (22.6298, 132) construction
  line L349 (22.6298, 132) -> (15.6298, 132) construction
  line L350 (15.6298, 132) -> (15.6298, 122) construction
  line L351 (15.6298, 122) -> (22.6298, 122) construction
  line L352 (22.6298, 137) -> (22.6298, 147) construction
  line L353 (22.6298, 147) -> (15.6298, 147) construction
  line L354 (15.6298, 147) -> (15.6298, 137) construction
  line L355 (15.6298, 137) -> (22.6298, 137) construction
  line L356 (22.6298, 152) -> (22.6298, 162) construction
  line L357 (22.6298, 162) -> (15.6298, 162) construction
  line L358 (15.6298, 162) -> (15.6298, 152) construction
  line L359 (15.6298, 152) -> (22.6298, 152) construction
  line L360 (22.6298, 167) -> (22.6298, 177) construction
  line L361 (22.6298, 177) -> (15.6298, 177) construction
  line L362 (15.6298, 177) -> (15.6298, 167) construction
  line L363 (15.6298, 167) -> (22.6298, 167) construction
  line L364 (22.6298, 182) -> (22.6298, 192) construction
  line L365 (22.6298, 192) -> (15.6298, 192) construction
  line L366 (15.6298, 192) -> (15.6298, 182) construction
  line L367 (15.6298, 182) -> (22.6298, 182) construction
  line L368 (10.6298, 2) -> (10.6298, 12) construction
  line L369 (10.6298, 12) -> (3.6298, 12) construction
  line L370 (3.6298, 12) -> (3.6298, 2) construction
  line L371 (3.6298, 2) -> (10.6298, 2) construction
  line L372 (10.6298, 17) -> (10.6298, 27) construction
  line L373 (10.6298, 27) -> (3.6298, 27) construction
  line L374 (3.6298, 27) -> (3.6298, 17) construction
  line L375 (3.6298, 17) -> (10.6298, 17) construction
  line L376 (10.6298, 32) -> (10.6298, 42) construction
  line L377 (10.6298, 42) -> (3.6298, 42) construction
  line L378 (3.6298, 42) -> (3.6298, 32) construction
  line L379 (3.6298, 32) -> (10.6298, 32) construction
  line L380 (10.6298, 47) -> (10.6298, 57) construction
  line L381 (10.6298, 57) -> (3.6298, 57) construction
  line L382 (3.6298, 57) -> (3.6298, 47) construction
  line L383 (3.6298, 47) -> (10.6298, 47) construction
  line L384 (10.6298, 62) -> (10.6298, 72) construction
  line L385 (10.6298, 72) -> (3.6298, 72) construction
  line L386 (3.6298, 72) -> (3.6298, 62) construction
  line L387 (3.6298, 62) -> (10.6298, 62) construction
  line L388 (10.6298, 77) -> (10.6298, 87) construction
  line L389 (10.6298, 87) -> (3.6298, 87) construction
  line L390 (3.6298, 87) -> (3.6298, 77) construction
  line L391 (3.6298, 77) -> (10.6298, 77) construction
  line L392 (10.6298, 92) -> (10.6298, 102) construction
  line L393 (10.6298, 102) -> (3.6298, 102) construction
  line L394 (3.6298, 102) -> (3.6298, 92) construction
  line L395 (3.6298, 92) -> (10.6298, 92) construction
  line L396 (10.6298, 107) -> (10.6298, 117) construction
  line L397 (10.6298, 117) -> (3.6298, 117) construction
  line L398 (3.6298, 117) -> (3.6298, 107) construction
  line L399 (3.6298, 107) -> (10.6298, 107) construction
  line L400 (10.6298, 122) -> (10.6298, 132) construction
  line L401 (10.6298, 132) -> (3.6298, 132) construction
  line L402 (3.6298, 132) -> (3.6298, 122) construction
  line L403 (3.6298, 122) -> (10.6298, 122) construction
  line L404 (10.6298, 137) -> (10.6298, 147) construction
  line L405 (10.6298, 147) -> (3.6298, 147) construction
  line L406 (3.6298, 147) -> (3.6298, 137) construction
  line L407 (3.6298, 137) -> (10.6298, 137) construction
  line L408 (10.6298, 152) -> (10.6298, 162) construction
  line L409 (10.6298, 162) -> (3.6298, 162) construction
  line L410 (3.6298, 162) -> (3.6298, 152) construction
  line L411 (3.6298, 152) -> (10.6298, 152) construction
  line L412 (99.6298, 2) -> (99.6298, 12) construction
  line L413 (99.6298, 12) -> (92.6298, 12) construction
  line L414 (92.6298, 12) -> (92.6298, 2) construction
  line L415 (92.6298, 2) -> (99.6298, 2) construction
  line L416 (85.6298, 17) -> (85.6298, 27) construction
  line L417 (85.6298, 27) -> (78.6298, 27) construction
  line L418 (78.6298, 27) -> (78.6298, 17) construction
  line L419 (78.6298, 17) -> (85.6298, 17) construction
  line L420 (99.6298, 17) -> (99.6298, 27) construction
  line L421 (99.6298, 27) -> (92.6298, 27) construction
  line L422 (92.6298, 27) -> (92.6298, 17) construction
  line L423 (92.6298, 17) -> (99.6298, 17) construction
  line L424 (99.6298, 32) -> (99.6298, 42) construction
  line L425 (99.6298, 42) -> (92.6298, 42) construction
  line L426 (92.6298, 42) -> (92.6298, 32) construction
  line L427 (92.6298, 32) -> (99.6298, 32) construction
  line L428 (99.6298, 47) -> (99.6298, 57) construction
  line L429 (99.6298, 57) -> (92.6298, 57) construction
  line L430 (92.6298, 57) -> (92.6298, 47) construction
  line L431 (92.6298, 47) -> (99.6298, 47) construction
  line L432 (99.6298, 62) -> (99.6298, 72) construction
  line L433 (99.6298, 72) -> (92.6298, 72) construction
  line L434 (92.6298, 72) -> (92.6298, 62) construction
  line L435 (92.6298, 62) -> (99.6298, 62) construction
  line L436 (99.6298, 77) -> (99.6298, 87) construction
  line L437 (99.6298, 87) -> (92.6298, 87) construction
  line L438 (92.6298, 87) -> (92.6298, 77) construction
  line L439 (92.6298, 77) -> (99.6298, 77) construction
  line L440 (99.6298, 92) -> (99.6298, 102) construction
  line L441 (99.6298, 102) -> (92.6298, 102) construction
  line L442 (92.6298, 102) -> (92.6298, 92) construction
  line L443 (92.6298, 92) -> (99.6298, 92) construction
  line L444 (99.6298, 107) -> (99.6298, 117) construction
  line L445 (99.6298, 117) -> (92.6298, 117) construction
  line L446 (92.6298, 117) -> (92.6298, 107) construction
  line L447 (92.6298, 107) -> (99.6298, 107) construction
  line L448 (85.6298, 32) -> (85.6298, 42) construction
  line L449 (85.6298, 42) -> (78.6298, 42) construction
  line L450 (78.6298, 42) -> (78.6298, 32) construction
  line L451 (78.6298, 32) -> (85.6298, 32) construction
  line L452 (85.6298, 47) -> (85.6298, 57) construction
  line L453 (85.6298, 57) -> (78.6298, 57) construction
  line L454 (78.6298, 57) -> (78.6298, 47) construction
  line L455 (78.6298, 47) -> (85.6298, 47) construction
  line L456 (85.6298, 62) -> (85.6298, 72) construction
  line L457 (85.6298, 72) -> (78.6298, 72) construction
  line L458 (78.6298, 72) -> (78.6298, 62) construction
  line L459 (78.6298, 62) -> (85.6298, 62) construction
  line L460 (85.6298, 77) -> (85.6298, 87) construction